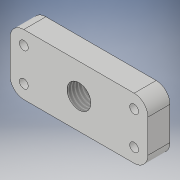
# Autodesk Inventor part: Part1
Saved by Autodesk Inventor 2019.4 (Build 234330000, 330)
## iProperties
Created: 2021-12-20
Part Number: Part1
Material: 一般
Document SubType Name: Modeling
Designer: 堀川皓史
Density: 1 g/cm^3
Appearance: 既定
Author: 堀川皓史
Autodesk Inventor part; units mm, degrees
ref_plane "YZ Plane" through (0, 0, 0) normal (1, 0, 0) x (0, 1, 0)
ref_plane "XZ Plane" through (0, 0, 0) normal (0, 1, 0) x (-1, 0, 0)
ref_plane "XY Plane" through (0, 0, 0) normal (0, 0, 1) x (1, 0, 0)
sketch "スケッチ1" plane through (0, 0, 0) normal (0, 0, 1) x (1, 0, 0)
  line L0 (25, 11) -> (-25, 11)
  line L1 (-25, 11) -> (-25, -11)
  line L2 (-25, -11) -> (25, -11)
  line L3 (25, -11) -> (25, 11)
  line L4 (25, 11) -> (-25, -11) construction
  line L5 (-25, 11) -> (25, -11) construction
  circle A0 centre (-20, 6) radius 1.6
  circle A1 centre (-20, -6) radius 1.6
  circle A2 centre (20, 6) radius 1.6
  circle A3 centre (20, -6) radius 1.6
  point P0 (0, 0)
  dimension "d0" = 50
  dimension "d1" = 22
  dimension "d14" = 3.2
  dimension "d15" = 3.2
  dimension "d16" = 3.2
  dimension "d17" = 3.2
  dimension "d18" = 40
  dimension "d19" = 5
  dimension "d20" = 12
  dimension "d21" = 5
  constraints: 12 end point, 4 centre point, 2 horizontal alignment, 2 midpoint, 2 parallel, 2 vertical alignment, 1 horizontal, 1 perpendicular
  measures "d0" distance of L2.end L1.end
  measures "d1" distance of L1.end L0.end
  measures "d14" diameter of A0
  measures "d15" diameter of A1
  measures "d16" diameter of A2
  measures "d17" diameter of A3
  measures "d18" distance of A3.centre A1.centre
  measures "d19" distance from line of L1 A1.centre
  measures "d20" distance of A0.centre A1.centre
  measures "d21" distance from line of L0 A0.centre
extrude "押し出し1" add sketch "スケッチ1" along normal blind 8
sketch "スケッチ2" plane through (0, 0, 8) normal (0, 0, 1) x (1, 0, 0)
  circle A0 centre (0, 0) radius 5
  dimension "d4" = 10
  constraints: 2 coincident, 1 centre point
  measures "d4" diameter of A0
hole "穴1" at (0, 0, 8) direction (0, 0, -1) diameter 8.647 end through all thread size "M10x1.25" class "6H" standard "ANSI Metric M Profile"
fillet "フィレット1" radius 5 4 edges at (25, 11, 4) (25, -11, 4) (-25, 11, 4) (-25, -11, 4)
